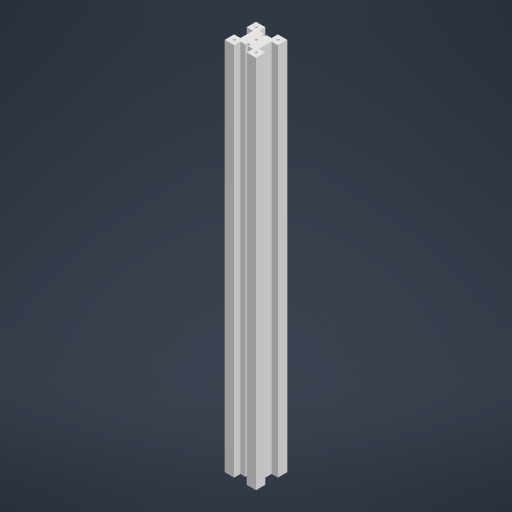
# Autodesk Inventor part: 1_inner_leg
Saved by Autodesk Inventor 2024 (Build 280153000, 153)
## iProperties
Created: 2023-05-22
Part Number: 1_inner_leg
Material: Generic
Document SubType Name: Modeling
Designer: aasmu
Density: 1 g/cm^3
Appearance: Default
width: 50.000 mm
rail_depth: 10.000 mm
rail_width: 20.000 mm
cabel_channel_depth: 4.000 mm
screw_hole_diameter: 4.000 mm
hole_spacing: 35.000 mm
cabel_channel_width: 4.000 mm
height: 600.000 mm
Author: aasmu
Autodesk Inventor part; units mm, degrees
ref_plane "YZ Plane" through (0, 0, 0) normal (1, 0, 0) x (0, 1, 0)
ref_plane "XZ Plane" through (0, 0, 0) normal (0, 1, 0) x (-1, 0, 0)
ref_plane "XY Plane" through (0, 0, 0) normal (0, 0, 1) x (1, 0, 0)
sketch "Sketch3" plane through (0, 0, 0) normal (0, 1, 0) x (-1, 0, 0)
  line L0 (0, 0) -> (0, -15)
  line L1 (-10, -15) -> (-10, -35)
  line L2 (-10, -35) -> (0, -35)
  line L3 (0, -15) -> (-10, -15)
  line L4 (0, -35) -> (0, -50)
  line L5 (0, -50) -> (-15, -50)
  line L6 (-15, -50) -> (-15, -40)
  line L7 (-15, -40) -> (-35, -40)
  line L8 (-35, -40) -> (-35, -50)
  line L9 (-35, -50) -> (-50, -50)
  line L10 (-50, -50) -> (-50, -35)
  line L11 (-50, -35) -> (-40, -35)
  line L12 (-40, -35) -> (-40, -15)
  line L13 (-40, -15) -> (-50, -15)
  line L14 (-50, -15) -> (-50, 0)
  line L15 (-50, 0) -> (-35, 0)
  line L16 (-35, 0) -> (-35, -10.0399)
  line L17 (-35, -10) -> (-15, -10)
  line L18 (-15, -10) -> (-15, 0)
  line L19 (-15, 0) -> (0, 0)
  line L20 (-23, -10) -> (-23, -14)
  line L21 (-23, -14) -> (-27, -14)
  line L22 (-23, -40) -> (-23, -36)
  line L23 (-23, -36) -> (-27, -36)
  line L24 (-27, -36) -> (-27, -40.4219)
  line L25 (-27, -14) -> (-27, -10)
  line L26 (-25, -40) -> (-25, -36) construction
  point P0 (-34.3495, -10)
  point P1 (-25, -14)
  point P2 (-35, -10)
  point P3 (-27, -40)
  dimension "width" = 50
  dimension "rail_depth" = 10
  dimension "rail_width" = 20
  dimension "cabel_channel_depth" = 4
  dimension "cabel_channel_width" = 4
  constraints: 54 end point, 17 equal length, 15 perpendicular, 7 vertical, 5 horizontal, 5 point on line, 3 midpoint, 1 coincident, 1 collinear
  measures "width" distance of L4.end L0.start
  measures "rail_depth" distance of L17.end L18.end
  measures "rail_width" distance of L17.start L17.end
  measures "cabel_channel_depth" distance of L22.start L22.end
  measures "cabel_channel_width" distance of L22.end L23.end
extrude "Extrusion3" add sketch "Sketch3" along normal blind 600 contours L0 L3 L1 L2 L4 L5 L6 L7 L22 L23 L24 L8 L9 L10 L11 L12 L13 L14 L15 L16 L17 L25 L21 L20 L18 L19
sketch "Sketch4" plane through (0, 600, 0) normal (0, 1, 0) x (1, 0, 0)
  line L0 (15, 50) -> (0, 50) projected
  line L1 (7.5, 50) -> (7.5, 35)
  line L2 (0, 35) -> (10, 35) projected
  line L3 (10, 35) -> (10, 15) projected
  line L4 (10, 25) -> (40, 25)
  line L5 (40, 15) -> (40, 35) projected
  circle A0 centre (7.5, 42.5) radius 2
  circle A1 centre (25, 25) radius 2
  circle A2 centre (42.5, 42.5) radius 2
  circle A3 centre (7.5, 7.5) radius 2
  circle A4 centre (42.5, 7.5) radius 2
  point P0 (0, 0)
  point P1 (27, 25)
  point P2 (23, 25)
  dimension "d22" = 4
  dimension "screw_hole_diameter" = 4
  dimension "hole_spacing" = 35
  dimension "d29" = 35
  constraints: 5 centre point, 5 midpoint, 4 end point, 2 coincident, 2 vertical, 1 horizontal, 1 point on line, 6 other
  measures "d22" diameter of A0
  measures "screw_hole_diameter" diameter of A1
  measures "hole_spacing" distance of A0.centre A2.centre
  measures "d29" distance of A0.centre A3.centre
extrude "Extrusion4" cut sketch "Sketch4" against normal blind 30
extrude "Extrusion5" cut sketch "Sketch4" along normal blind 30 from surface at -600
equation "\"hole_spacing\" = 0.5 * width + 0.5 * rail_width"
equation "\"d34\" = hole_depth"
equation "\"hole_depth\" = 30"
body "Solid2"
